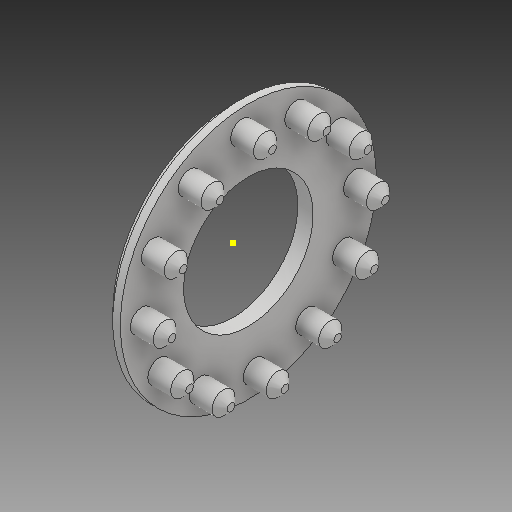
# Autodesk Inventor part: Servoscheibenflansch
Saved by Autodesk Inventor 2018 (Build 220112000, 112)
## iProperties
Part Number: Servoscheibenflansch
Material: Generisch
Document SubType Name: Modeling
Designer: Jochen Alt
Density: 1 g/cm^3
Appearance: Vorgabe
Mass: 0.195373 g
Surface Area: 4.86181 cm^2
Volume: 0.195373 cm^3
Author: Jochen Alt
Autodesk Inventor part; units mm, degrees
ref_plane "YZ Plane" through (0, 0, 0) normal (1, 0, 0) x (0, 1, 0)
ref_plane "XZ Plane" through (0, 0, 0) normal (0, 1, 0) x (-1, 0, 0)
ref_plane "XY Plane" through (0, 0, 0) normal (0, 0, 1) x (1, 0, 0)
sketch "Skizze1" plane through (0, 0, 0) normal (0, 0, 1) x (1, 0, 0)
  point P0 (0, 0)
sketch "Skizze2" plane through (0, 0, 0) normal (1, 0, 0) x (0, 1, 0)
  circle A0 centre (0, 0) radius 8.4
  dimension "d0" = 16.8
  constraints: 1 centre point, 1 coincident
  measures "d0" diameter of A0
extrude "Extrusion1" add sketch "Skizze2" along normal blind 1
sketch "Skizze3" plane through (1, 0, 0) normal (1, 0, 0) x (0, 0, -1)
  circle A0 centre (0, 0) radius 8.4 projected
  circle A1 centre (-0.4149, 7) radius 0.75
  dimension "d3" = 1.5
  dimension "d4" = 7
  constraints: 1 centre point
  measures "d3" diameter of A1
  measures "d4" vertical distance of A0.centre A1.centre
extrude "Extrusion2" add sketch "Skizze3" along normal blind 2 contours A1
chamfer "Fase1" distance 0.5 angle 45 1 edges at (3, 7, 1.1649)
pattern_circular "Runde Anordnung1" count 12 over 360 about axis through (0, 0, 0) along (1, 0, 0) of "Extrusion2", "Fase1"
sketch "Skizze4" plane through (1, 0, 0) normal (1, 0, 0) x (0, 0, -1)
  circle A0 centre (0, 0) radius 8.4 projected
  circle A1 centre (0, 0) radius 4.25
  dimension "d16" = 8.5
  constraints: 1 centre point, 1 coincident
  measures "d16" diameter of A1
extrude "Extrusion3" cut sketch "Skizze4" against normal up to next contours A1
chamfer "Fase3" distance 0.5 angle 45 1 edges at (0, -8.4, 0)
